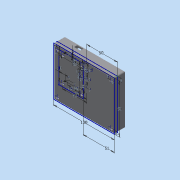
# Autodesk Inventor part: Base_V2
Saved by Autodesk Inventor 2015 (Build 190159000, 159)
## iProperties
Created: 2014-12-24
Part Number: Base_V2
Material: Generic
Document SubType Name: Modeling
Designer: Openlab
Density: 1 g/cm^3
Appearance: Default
Author: Openlab
Autodesk Inventor part; units mm, degrees
ref_plane "YZ Plane" through (0, 0, 0) normal (1, 0, 0) x (0, 1, 0)
ref_plane "XZ Plane" through (0, 0, 0) normal (0, 1, 0) x (-1, 0, 0)
ref_plane "XY Plane" through (0, 0, 0) normal (0, 0, 1) x (1, 0, 0)
sketch "Sketch1" plane through (0, 0, 0) normal (0, 1, 0) x (-1, 0, 0)
  line L0 (100, 0) -> (0, 0)
  line L1 (0, 0) -> (0, -80)
  line L2 (0, -80) -> (100, -80)
  line L3 (100, -80) -> (100, 0)
  line L4 (95, -5) -> (77, -5)
  line L5 (5, -5) -> (5, -75)
  line L6 (5, -75) -> (95, -75)
  line L7 (95, -75) -> (95, -5)
  line L8 (37.7, -8.55) -> (24.7, -8.55)
  line L9 (24.7, -8.55) -> (24.7, -21.55)
  line L10 (24.7, -21.55) -> (37.7, -21.55)
  line L11 (95, -65) -> (95, -5)
  line L12 (37.7, -48.55) -> (24.7, -48.55)
  line L13 (24.7, -48.55) -> (24.7, -61.55)
  line L14 (24.7, -61.55) -> (37.7, -61.55)
  line L15 (95, -5) -> (90, -5)
  line L16 (90, -5) -> (90, -10)
  line L17 (90, -10) -> (95, -10)
  line L18 (95, -10) -> (95, -5)
  line L19 (95, -75) -> (90, -75)
  line L20 (90, -75) -> (90, -70)
  line L21 (90, -70) -> (95, -70)
  line L22 (95, -70) -> (95, -75)
  line L23 (5, -5) -> (10, -5)
  line L24 (10, -5) -> (10, -10)
  line L25 (10, -10) -> (5, -10)
  line L26 (5, -10) -> (5, -5)
  line L27 (5, -75) -> (10, -75)
  line L28 (10, -75) -> (10, -70)
  line L29 (10, -70) -> (5, -70)
  line L30 (5, -70) -> (5, -75)
  line L31 (77, -5) -> (77, -2.55)
  line L32 (77, -2.55) -> (67, -2.55)
  line L33 (67, -2.55) -> (67, -5)
  line L34 (77, -5) -> (72.2264, -5) construction
  line L35 (95, -5) -> (77, -5)
  line L36 (72.2264, -5) -> (67, -5) construction
  line L37 (67, -5) -> (55.2, -5)
  line L38 (14.7, -65) -> (14.7, -5)
  line L39 (42.7, -65) -> (14.7, -65)
  line L40 (14.7, -5) -> (5, -5)
  line L41 (39.55, -60.05) -> (40.85, -60.05)
  line L42 (40.85, -50.05) -> (39.55, -50.05)
  line L43 (37.7, -56.55) -> (39.55, -56.55)
  line L44 (40.85, -56.55) -> (42.7, -56.55)
  line L45 (42.7, -53.55) -> (40.85, -53.55)
  line L46 (39.55, -53.55) -> (37.7, -53.55)
  line L47 (39.55, -40.05) -> (40.85, -40.05)
  line L48 (40.85, -30.05) -> (39.55, -30.05)
  line L49 (42.7, -36.55) -> (40.85, -36.55)
  line L50 (39.55, -36.55) -> (37.7, -36.55)
  line L51 (42.7, -33.55) -> (40.85, -33.55)
  line L52 (39.55, -33.55) -> (37.7, -33.55)
  line L53 (38.65, -20.05) -> (41.75, -20.05)
  line L54 (41.75, -10.05) -> (38.65, -10.05)
  line L55 (37.7, -16.55) -> (38.65, -16.55)
  line L56 (41.75, -16.55) -> (42.7, -16.55)
  line L57 (37.7, -13.55) -> (38.65, -13.55)
  line L58 (41.75, -13.55) -> (42.7, -13.55)
  line L59 (14.7, -57.55) -> (24.7, -57.55)
  line L60 (14.7, -52.55) -> (24.7, -52.55)
  line L61 (14.7, -37.55) -> (24.7, -37.55)
  line L62 (14.7, -32.55) -> (24.7, -32.55)
  line L63 (14.7, -17.55) -> (24.7, -17.55)
  line L64 (14.7, -12.55) -> (24.7, -12.55)
  line L65 (44.4, -5) -> (44.4, -65)
  line L66 (67, -5) -> (47.4, -5)
  line L67 (44.4, -5) -> (42.7, -5)
  line L68 (41.4, -75) -> (41.4, -72)
  line L69 (44.4, -5) -> (47.4, -5)
  line L70 (13, -5) -> (13, -72)
  line L71 (13, -72) -> (14.7, -72)
  line L72 (10, -70) -> (10, -5)
  line L73 (14.7, -72) -> (14.7, -75)
  line L74 (2.55, -77.45) -> (2.55, -2.55)
  line L75 (2.55, -2.55) -> (97.45, -2.55)
  line L76 (97.45, -2.55) -> (97.45, -77.45)
  line L77 (97.45, -77.45) -> (2.55, -77.45)
  line L78 (44.4, -65) -> (47.4, -65)
  line L79 (47.4, -75) -> (47.4, -72)
  line L80 (47.4, -65) -> (47.4, -5)
  line L81 (47.4, -72) -> (41.4, -72)
  line L82 (42.1668, -15.05) -> (13.95, -15.05) construction
  line L83 (37.7, -8.55) -> (37.7, -21.55)
  line L84 (40.2, -5.5957) -> (40.2, -61.9523) construction
  line L85 (41.75, -10.05) -> (41.75, -20.05)
  line L86 (38.65, -10.05) -> (38.65, -20.05)
  line L87 (44.1467, -35.05) -> (11.3232, -35.05) construction
  line L88 (40.85, -30.05) -> (40.85, -40.05)
  line L89 (39.55, -30.05) -> (39.55, -40.05)
  line L90 (13.6727, -55.05) -> (43.8542, -55.05) construction
  line L91 (40.85, -50.05) -> (40.85, -60.05)
  line L92 (39.55, -50.05) -> (39.55, -60.05)
  line L93 (42.7, -5) -> (42.7, -65)
  line L94 (37.7, -48.55) -> (37.7, -61.55)
  line L95 (37.7, -28.55) -> (24.7, -28.55)
  line L96 (24.7, -28.55) -> (24.7, -41.55)
  line L97 (24.7, -41.55) -> (37.7, -41.55)
  line L98 (37.7, -41.55) -> (37.7, -28.55)
  dimension "d1" = 5
  dimension "d2" = 5
  dimension "d3" = 5
  dimension "d4" = 5
  dimension "d32" = 13
  dimension "d36" = 70
  dimension "d55" = 5
  dimension "d56" = 5
  dimension "d57" = 5
  dimension "d58" = 5
  dimension "d59" = 5
  dimension "d60" = 5
  dimension "d61" = 5
  dimension "d62" = 5
  dimension "d186" = 10
  dimension "d187" = 90
  dimension "d197" = 80
  dimension "d234" = 1.3
  dimension "d235" = 10
  dimension "d253" = 3
  dimension "d254" = 1.3
  dimension "d255" = 10
  dimension "d265" = 3
  dimension "d266" = 3.1
  dimension "d267" = 10
  dimension "d273" = 5
  dimension "d275" = 5
  dimension "d277" = 5
  dimension "d297" = 10
  dimension "d298" = 60
  dimension "d306" = 3
  dimension "d364" = 23
  dimension "d371" = 2.55
  dimension "d372" = 2.55
  dimension "d373" = 2.55
  dimension "d374" = 2.55
  dimension "d386" = 3
  dimension "d387" = 6
  dimension "d391" = 3
  dimension "d395" = 13
  dimension "d400" = 12.5
  dimension "d401" = 20
  dimension "d402" = 20
  dimension "d405" = 13
  dimension "d406" = 5
  dimension "d407" = 1.7
  dimension "d408" = 3
  dimension "d410" = 13
  dimension "d440" = 3
  dimension "d441" = 1.7
  constraints: 198 end point, 42 point on line, 34 perpendicular, 31 parallel, 26 horizontal, 16 collinear, 9 vertical, 1 coincident, 16 other
  measures "d1" distance between parallel lines of L2 L6
  measures "d2" distance between parallel lines of L7 L3
  measures "d3" distance between parallel lines of L1 L5
  measures "d4" distance between parallel lines of L4 L0
  measures "d32" distance of L14.end L12.start
  measures "d36" distance of L5.start L5.end
  measures "d55" distance of L17.end L16.end
  measures "d56" distance of L16.end L15.end
  measures "d57" distance of L20.end L21.end
  measures "d58" distance of L19.end L20.end
  measures "d59" distance of L24.end L25.end
  measures "d60" distance of L23.end L24.end
  measures "d61" distance of L29.end L28.end
  measures "d62" distance of L28.end L27.end
  measures "d186" distance of L31.end L32.end
  measures "d187" distance of L5.end L6.end
  measures "d197" distance between parallel lines of L0 L2
  measures "d234" distance of L42.start L42.end
  measures "d235" distance of L41.end L42.start
  measures "d253" distance between parallel lines of L46 L43
  measures "d254" distance of L48.end L48.start
  measures "d255" distance of L48.start L47.end
  measures "d265" distance between parallel lines of L51 L49
  measures "d266" distance of L54.end L54.start
  measures "d267" distance of L54.start L53.end
  measures "d273" distance between parallel lines of L64 L63
  measures "d275" distance between parallel lines of L62 L61
  measures "d277" distance between parallel lines of L59 L60
  measures "d297" distance between parallel lines of L13 L38
  measures "d298" distance of L38.start L38.end
  measures "d306" distance of L68.start L68.end
  measures "d364" distance between parallel lines of L3 L31
  measures "d371" distance between parallel lines of L1 L74
  measures "d372" distance between parallel lines of L0 L75
  measures "d373" distance between parallel lines of L2 L77
  measures "d374" distance between parallel lines of L3 L76
  measures "d386" distance of L65.end L78.end
  measures "d387" distance of L79.end L68.end
  measures "d391" distance of L71.end L73.end
  measures "d395" distance between parallel lines of L10 L8
  measures "d400" distance between parallel lines of L82 L75
  measures "d401" distance between parallel lines of L87 L82
  measures "d402" distance between parallel lines of L90 L87
  measures "d405" distance between parallel lines of L13 L94
  measures "d406" distance between parallel lines of L94 L93
  measures "d407" distance between parallel lines of L93 L65
  measures "d408" distance between parallel lines of L55 L57
  measures "d410" distance between parallel lines of L97 L95
  measures "d440" distance between parallel lines of L72 L70
  measures "d441" distance between parallel lines of L70 L38
extrude "Extrusion1" add sketch "Sketch1" against normal blind 5 contours L3 L2 L1 L0 | L7 L17 L16 L4 | L4 L31 L75 L76 L77 L74 L33 L37 L66 L69 L67 L93 L58 L85 L54 L86 L57 L83 L8 L9 L64 L38 L40 L23 L5 L6 L7 | L16 L17 L7 L21 L20 L6 L79 L81 L68 L73 L71 L70 L40 L38 L39 L93 L67 L65 L78 L80 L66 L37 L33 L32 L31 L4 | L7 L6 L20 L21 | L6 L68 L81 L79 | L80 L78 L65 L69 | L6 L28 L72 L24 L40 L70 L71 L73 | L6 L5 L29 L28 | L93 L56 L85 L58 | L29 L5 L25 L72 | L85 L53 L86 L54 | L93 L51 L88 L48 L89 L52 L98 L95 L96 L62 L38 L63 L9 L10 L83 L55 L86 L53 L85 L56 | L25 L5 L23 L24 | L93 L49 L88 L51 | L88 L47 L89 L48 | L93 L45 L91 L42 L92 L46 L94 L12 L13 L60 L38 L61 L96 L97 L98 L50 L89 L47 L88 L49 | L64 L9 L63 L38 | L86 L55 L83 L57 | L93 L44 L91 L45 | L9 L8 L83 L10 | L91 L41 L92 L42 | L93 L39 L38 L59 L13 L14 L94 L43 L92 L41 L91 L44 | L62 L96 L61 L38 | L89 L50 L98 L52 | L96 L95 L98 L97 | L60 L13 L59 L38 | L92 L43 L94 L46 | L13 L12 L94 L14
sketch "Sketch3" plane through (0, 0, 0) normal (0, 1, 0) x (-1, 0, 0)
  line L0 (50, -5) -> (50, -55)
  line L1 (90, -55) -> (90, -5)
  line L2 (90, -5) -> (50, -5)
  line L3 (50, -55) -> (90, -55)
  line L4 (81.271, -5) -> (62.729, -5)
  line L5 (62.729, -5) -> (62.729, -48.18)
  line L6 (62.729, -48.18) -> (81.271, -48.18)
  line L7 (81.271, -48.18) -> (81.271, -5)
  line L8 (72, 1.7089) -> (72, -57.768) construction
  line L9 (76, -10) -> (68, -10)
  line L10 (68, -10) -> (68, -5)
  line L11 (68, -5) -> (76, -5)
  line L12 (76, -5) -> (76, -10)
  circle A0 centre (86, -50) radius 3.5
  circle A1 centre (55, -50) radius 3.5
  circle A2 centre (86, -10) radius 3.5
  circle A3 centre (55, -10) radius 3.5
  line L13 (60.5, -21.25) -> (58, -21.25)
  line L14 (58, -21.25) -> (58, -31.25)
  line L15 (58, -31.25) -> (60.5, -31.25)
  line L16 (60.5, -31.25) -> (60.5, -21.25)
  line L17 (55.5, -21.25) -> (53, -21.25)
  line L18 (53, -21.25) -> (53, -38.75)
  line L19 (53, -38.75) -> (55.5, -38.75)
  line L20 (55.5, -38.75) -> (55.5, -21.25)
  point P0 (0, 0)
  dimension "d37" = 40
  dimension "d38" = 50
  dimension "d39" = 5
  dimension "d40" = 4
  dimension "d41" = 5
  dimension "d42" = 5
  dimension "d43" = 18.542
  dimension "d44" = 43.18
  dimension "d45" = 8
  dimension "d46" = 5
  dimension "d47" = 50
  dimension "d48" = 5
  dimension "d119" = 22
  dimension "d148" = 7
  dimension "d149" = 7
  dimension "d150" = 7
  dimension "d151" = 7
  dimension "d433" = 2.5
  dimension "d434" = 10
  dimension "d435" = 2.5
  dimension "d436" = 17.5
  dimension "d437" = 16.25
  dimension "d438" = 3
  dimension "d439" = 2.5
  constraints: 42 end point, 10 parallel, 5 coincident, 5 horizontal, 5 perpendicular, 4 centre point, 4 horizontal alignment, 2 vertical alignment, 1 collinear, 1 vertical, 2 other
  measures "d37" distance of L1.start L0.end
  measures "d38" distance of L1.end L1.start
  measures "d39" distance from line of L2 point (86, -10)
  measures "d40" distance from line of L1 point (86, -50)
  measures "d41" distance from line of L3 point (86, -50)
  measures "d42" distance from line of L0 point (55, -10)
  measures "d43" distance of L5.end L6.end
  measures "d44" distance of L4.end L5.end
  measures "d45" distance of L9.start L9.end
  measures "d46" distance of L11.end L9.start
  measures "d47" distance from line of point (0, 0) L0
  measures "d48" vertical distance of point (0, 0) point (50, -5)
  measures "d119" distance between parallel lines of L8 L0
  measures "d148" diameter of A0
  measures "d149" diameter of A1
  measures "d150" diameter of A2
  measures "d151" diameter of A3
  measures "d433" distance of L15.end L14.end
  measures "d434" distance of L14.end L13.end
  measures "d435" distance of L20.start L19.start
  measures "d436" distance of L19.start L17.end
  measures "d437" distance between parallel lines of L17 L2
  measures "d438" distance between parallel lines of L0 L18
  measures "d439" distance between parallel lines of L20 L14
extrude "Extrusion4" add sketch "Sketch3" along normal blind 2 contours A0 | A1 | A2 | A3
sketch "Sketch5" plane through (0, -5, 0) normal (0, -1, 0) x (1, 0, 0)
  line L0 (-100, 0) -> (0, 0)
  line L1 (0, 0) -> (0, -80)
  line L2 (0, -80) -> (-100, -80)
  line L3 (-100, -80) -> (-100, 0)
  line L4 (-51, -5) -> (-51, -55)
  line L5 (-91, -55) -> (-91, -5)
  line L6 (-51, -55) -> (-91, -55)
  line L7 (-91, -5) -> (-51, -5)
  point P0 (-94, -74)
  point P1 (-94, -6)
  point P2 (-6, -6)
  point P3 (-6, -74)
  point P4 (-55, -10)
  point P5 (-86, -10)
  point P6 (-86, -50)
  point P7 (-55, -50)
  dimension "d310" = 100
  dimension "d311" = 80
  dimension "d314" = 6
  dimension "d315" = 6
  dimension "d316" = 6
  dimension "d317" = 6
  dimension "d326" = 50
  dimension "d342" = 40
  dimension "d347" = 5
  dimension "d352" = 4
  dimension "d353" = 5
  dimension "d354" = 5
  dimension "d355" = 51
  dimension "d356" = 5
  constraints: 16 end point, 4 horizontal alignment, 4 parallel, 4 vertical alignment, 2 coincident, 2 perpendicular, 1 horizontal
  measures "d310" distance of L1.end L2.end
  measures "d311" distance of L0.end L1.end
  measures "d314" distance from line of L0 point (-6, -6)
  measures "d315" distance from line of L1 point (-6, -6)
  measures "d316" distance from line of L2 point (-6, -74)
  measures "d317" distance from line of L3 point (-94, -6)
  measures "d326" distance of L4.end L4.start
  measures "d342" distance of L5.end L4.start
  measures "d347" distance from line of L5 point (-86, -10)
  measures "d352" distance from line of L4 point (-55, -10)
  measures "d353" distance from line of L7 point (-55, -10)
  measures "d354" distance from line of L6 point (-55, -50)
  measures "d355" distance between parallel lines of L1 L4
  measures "d356" distance between parallel lines of L0 L7
hole "Hole22" at (-55, -5, -10) at (-86, -5, -10) at (-86, -5, -50) at (-55, -5, -50) direction (0, 1, 0) diameter 4 end through all counterbore diameter 6.5 counterbore depth 3
extrude "Extrusion16" add sketch "Sketch1" along normal blind 12.5
sketch "Sketch7" plane through (-100, -5, 0) normal (0, 0, 1) x (1, 0, 0)
  line L0 (23, 16) -> (33, 16)
  line L1 (33, 16) -> (33, 11)
  line L2 (33, 11) -> (23, 11)
  line L3 (23, 11) -> (23, 16)
  line L4 (0, 17.5) -> (0, 0) projected
  point P0 (100, 5)
  dimension "d380" = 10
  dimension "d381" = 5
  dimension "d382" = 23
  dimension "d383" = 11
  constraints: 8 end point, 2 parallel, 1 horizontal, 1 perpendicular
  measures "d380" distance of L1.end L2.end
  measures "d381" distance of L0.end L1.end
  measures "d382" distance between parallel lines of L4 L3
  measures "d383" distance from line of L4.end L2
extrude "Extrusion17" cut sketch "Sketch7" against normal blind 12.5
extrude "Extrusion19" add sketch "Sketch1" along normal blind 15 contours L7 L17 L16 L4 | L4 L31 L75 L76 L77 L74 L33 L37 L66 L69 L67 L93 L58 L85 L54 L86 L57 L83 L8 L9 L64 L38 L40 L23 L5 L6 L7 | L7 L6 L20 L21 | L6 L5 L29 L28 | L93 L51 L88 L48 L89 L52 L98 L95 L96 L62 L38 L63 L9 L10 L83 L55 L86 L53 L85 L56 | L25 L5 L23 L24 | L93 L45 L91 L42 L92 L46 L94 L12 L13 L60 L38 L61 L96 L97 L98 L50 L89 L47 L88 L49 | L93 L39 L38 L59 L13 L14 L94 L43 L92 L41 L91 L44
extrude "Extrusion20" add sketch "Sketch1" along normal blind 5 contours L93 L56 L85 L58 | L93 L49 L88 L51 | L64 L9 L63 L38 | L86 L55 L83 L57 | L93 L44 L91 L45 | L62 L96 L61 L38 | L89 L50 L98 L52 | L60 L13 L59 L38 | L92 L43 L94 L46
extrude "Extrusion21" add sketch "Sketch1" along normal blind 2.5 contours L85 L53 L86 L54 | L88 L47 L89 L48 | L91 L41 L92 L42
extrude "Extrusion22" add sketch "Sketch1" along normal blind 2.5 contours L6 L68 L81 L79 | L80 L78 L65 L69 | L6 L28 L72 L24 L40 L70 L71 L73
hole "Hole21" at (-6, -5, -6) at (-94, -5, -6) at (-94, -5, -74) at (-6, -5, -74) direction (0, 1, 0) diameter 4 end through all counterbore diameter 6.5 counterbore depth 3
fillet "Fillet4" radius 2.5 6 edges at (-19.7, 5, -57.55) (-19.7, 5, -52.55) (-19.7, 5, -37.55) (-19.7, 5, -32.55) (-19.7, 5, -17.55) (-19.7, 5, -12.55)
sketch "Sketch9" plane through (-14.7, 0, -5) normal (1, 0, 0) x (0, 0, -1)
  point P0 (-5, 0)
ref_plane "Work Plane1" through (-14.7, 0, -5) normal (1, 0, 0) x (0, 0, -1)
sketch "Sketch10" plane through (-14.7, -5, 0) normal (1, 0, 0) x (0, 0, -1)
  line L0 (80, 0) -> (0, 0) construction
  line L1 (0, 0) -> (0, 17.5) construction
  arc A0 (12, 12.5) -> (18, 12.5) centre (15, 12.5) ccw
  arc A1 (32, 12.5) -> (38, 12.5) centre (35, 12.5) ccw
  arc A2 (52, 12.5) -> (58, 12.5) centre (55, 12.5) ccw
  line L2 (12, 12.5) -> (12, 20)
  line L3 (12, 20) -> (18, 20)
  line L4 (18, 20) -> (18, 12.5)
  line L5 (32, 12.5) -> (32, 20)
  line L6 (32, 20) -> (38, 20)
  line L7 (38, 20) -> (38, 12.5)
  line L8 (52, 12.5) -> (52, 20)
  line L9 (52, 20) -> (58, 20)
  line L10 (58, 20) -> (58, 12.5)
  line L11 (65, 5) -> (65, 20) projected
  line L12 (57.55, 20) -> (65, 20) projected
  point P0 (0, 5)
  dimension "d423" = 20
  dimension "d424" = 20
  dimension "d425" = 6
  dimension "d426" = 6
  dimension "d427" = 6
  dimension "d431" = 7.5
  dimension "d432" = 10
  constraints: 18 end point, 6 point on circle, 6 tangent, 5 perpendicular, 3 centre point, 3 coincident, 2 collinear, 2 horizontal alignment, 2 point on line, 2 vertical, 1 parallel
  measures "d423" distance of point (35, 12.5) point (15, 12.5)
  measures "d424" distance of point (55, 12.5) point (35, 12.5)
  measures "d425" diameter of A0
  measures "d426" diameter of A1
  measures "d427" diameter of A2
  measures "d431" distance from line of L9 A2.centre
  measures "d432" distance from line of L11 point (55, 12.5)
extrude "Extrusion23" cut sketch "Sketch10" against normal blind 1.5
fillet "Fillet5" radius 2 8 edges at (0, 3.75, 0) (-100, 3.75, 0) (-100, 3.75, -80) (0, 3.75, -80) (-50, -5, -80) (0, -5, -40) (-50, -5, 0) (-100, -5, -40)
body "Solid1"
